Autodesk Inventor part; units mm, degrees
(part 2 of 2)
  spline S152 degree 2 poles (85.5825, 374.6714) (85.5825, 373.4202) (84.1936, 371.3057) (81.7162, 370.2172) (79.8144, 370.2172) knots 0 0 0 1 2 3 3 3 projected
  spline S153 degree 2 poles (79.8144, 370.2172) (76.4987, 370.2172) (73.9338, 372.7696) (73.7711, 374.7465) knots 0 0 0 1 2 2 2 projected
  line L321 (73.7711, 374.7465) -> (77.5998, 374.9842) projected
  spline S154 degree 2 poles (65.5507, 383.6676) (68.7913, 383.6676) (72.3072, 380.1767) (72.3072, 377.0362) knots 0 0 0 1 2 2 2 projected
  spline S155 degree 2 poles (72.3072, 377.0362) (72.3072, 374.759) (70.7682, 371.8437) (67.8654, 370.2172) (65.7008, 370.2172) knots 0 0 0 1 2 3 3 3 projected
  spline S156 degree 2 poles (65.7008, 370.2172) (63.5112, 370.2172) (60.621, 371.6185) (58.8317, 374.6589) (58.8317, 376.9361) knots 0 0 0 1 2 3 3 3 projected
  spline S157 degree 2 poles (58.8317, 376.9361) (58.8317, 380.1142) (62.3852, 383.6676) (65.5507, 383.6676) knots 0 0 0 1 2 2 2 projected
  line L322 (35.6094, 377.8495) -> (41.8154, 377.8495) projected
  line L323 (41.8154, 377.8495) -> (41.8154, 372.3192) projected
  spline S158 degree 2 poles (41.8154, 372.3192) (40.0262, 371.093) (37.286, 370.2172) (35.4092, 370.2172) knots 0 0 0 1 2 2 2 projected
  spline S159 degree 2 poles (35.4092, 370.2172) (33.0945, 370.2172) (30.1667, 371.7937) (28.5651, 374.9217) (28.5651, 376.9486) knots 0 0 0 1 2 3 3 3 projected
  spline S160 degree 2 poles (28.5651, 376.9486) (28.5651, 379.0757) (30.3168, 382.2162) (32.0185, 383.042) knots 0 0 0 1 2 2 2 projected
  spline S161 degree 2 poles (32.0185, 383.042) (33.3447, 383.6676) (35.5719, 383.6676) knots 0 0 0 1 1 1 projected
  spline S162 degree 2 poles (35.5719, 383.6676) (37.7365, 383.6676) (39.876, 382.8918) (41.2899, 381.2403) (41.6402, 379.9891) knots 0 0 0 1 2 3 3 3 projected
  line L324 (41.6402, 379.9891) -> (37.7615, 379.2884) projected
  spline S163 degree 2 poles (37.7615, 379.2884) (37.5238, 380.0266) (36.3726, 380.8148) (35.4843, 380.8148) knots 0 0 0 1 2 2 2 projected
  spline S164 degree 2 poles (35.4843, 380.8148) (34.1705, 380.8148) (32.594, 378.9756) (32.594, 376.9862) knots 0 0 0 1 2 2 2 projected
  spline S165 degree 2 poles (32.594, 376.9862) (32.594, 374.8841) (34.183, 373.0699) (35.6094, 373.0699) knots 0 0 0 1 2 2 2 projected
  spline S166 degree 2 poles (35.6094, 373.0699) (36.2851, 373.0699) (37.5112, 373.4578) (38.2995, 373.9332) knots 0 0 0 1 2 2 2 projected
  line L325 (38.2995, 373.9332) -> (38.2995, 375.1469) projected
  line L326 (38.2995, 375.1469) -> (35.6094, 375.1469) projected
  line L327 (35.6094, 375.1469) -> (35.6094, 377.8495) projected
  line L328 (8.9212, 383.4424) -> (15.6152, 383.4424) projected
  spline S167 degree 2 poles (15.6152, 383.4424) (17.467, 383.4424) (19.4439, 382.8043) (20.645, 381.0776) (20.645, 379.8389) knots 0 0 0 1 2 3 3 3 projected
  spline S168 degree 2 poles (20.645, 379.8389) (20.645, 378.7504) (19.7191, 377.1864) (18.9184, 376.6984) knots 0 0 0 1 2 2 2 projected
  spline S169 degree 2 poles (18.9184, 376.6984) (18.4054, 376.3856) (17.5045, 376.1854) knots 0 0 0 1 1 1 projected
  spline S170 degree 2 poles (17.5045, 376.1854) (18.2177, 375.9477) (18.5555, 375.7099) knots 0 0 0 1 1 1 projected
  spline S171 degree 2 poles (18.5555, 375.7099) (18.7682, 375.5473) (19.6065, 374.4963) (19.7567, 374.2085) knots 0 0 0 1 2 2 2 projected
  line L329 (19.7567, 374.2085) -> (21.696, 370.4424) projected
  line L330 (21.696, 370.4424) -> (17.1542, 370.4424) projected
  line L331 (17.1542, 370.4424) -> (15.0146, 374.4212) projected
  spline S172 degree 2 poles (15.0146, 374.4212) (14.6142, 375.1844) (14.3014, 375.4222) knots 0 0 0 1 1 1 projected
  spline S173 degree 2 poles (14.3014, 375.4222) (13.8635, 375.7225) (13.313, 375.7225) knots 0 0 0 1 1 1 projected
  line L332 (13.313, 375.7225) -> (12.9626, 375.7225) projected
  line L333 (12.9626, 375.7225) -> (12.9626, 370.4424) projected
  line L334 (12.9626, 370.4424) -> (8.9212, 370.4424) projected
  line L335 (8.9212, 370.4424) -> (8.9212, 383.4424) projected
  line L336 (-1.8516, 372.5944) -> (-2.4897, 370.4424) projected
  line L337 (-2.4897, 370.4424) -> (-6.5937, 370.4424) projected
  line L338 (-6.5937, 370.4424) -> (-1.7015, 383.4424) projected
  line L339 (-1.7015, 383.4424) -> (2.6903, 383.4424) projected
  line L340 (2.6903, 383.4424) -> (7.5699, 370.4424) projected
  line L341 (7.5699, 370.4424) -> (3.3659, 370.4424) projected
  line L342 (3.3659, 370.4424) -> (2.7153, 372.5944) projected
  line L343 (2.7153, 372.5944) -> (-1.8516, 372.5944) projected
  spline S174 degree 2 poles (-25.0114, 383.4424) (-23.1346, 383.4424) (-21.1201, 381.5781) (-21.1201, 380.2018) knots 0 0 0 1 2 2 2 projected
  spline S175 degree 2 poles (-21.1201, 380.2018) (-21.1201, 379.0507) (-21.8333, 378.2249) knots 0 0 0 1 1 1 projected
  spline S176 degree 2 poles (-21.8333, 378.2249) (-22.3213, 377.6743) (-23.2472, 377.349) knots 0 0 0 1 1 1 projected
  spline S177 degree 2 poles (-23.2472, 377.349) (-21.8458, 377.0112) (-20.5196, 375.3721) (-20.5196, 374.1334) knots 0 0 0 1 2 2 2 projected
  spline S178 degree 2 poles (-20.5196, 374.1334) (-20.5196, 373.1325) (-21.458, 371.5184) (-22.2712, 371.043) knots 0 0 0 1 2 2 2 projected
  spline S179 degree 2 poles (-22.2712, 371.043) (-22.7842, 370.7552) (-23.7977, 370.6175) knots 0 0 0 1 1 1 projected
  spline S180 degree 2 poles (-23.7977, 370.6175) (-25.1615, 370.4424) (-25.5994, 370.4424) knots 0 0 0 1 1 1 projected
  line L344 (-25.5994, 370.4424) -> (-32.5311, 370.4424) projected
  line L345 (-32.5311, 370.4424) -> (-32.5311, 383.4424) projected
  line L346 (-32.5311, 383.4424) -> (-25.0114, 383.4424) projected
  line L347 (-65.0999, 383.4424) -> (-60.1952, 376.248) projected
  line L348 (-60.1952, 376.248) -> (-60.1952, 383.4424) projected
  line L349 (-60.1952, 383.4424) -> (-56.4041, 383.4424) projected
  line L350 (-56.4041, 383.4424) -> (-56.4041, 370.4424) projected
  line L351 (-56.4041, 370.4424) -> (-60.1952, 370.4424) projected
  line L352 (-60.1952, 370.4424) -> (-65.0749, 377.5993) projected
  line L353 (-65.0749, 377.5993) -> (-65.0749, 370.4424) projected
  line L354 (-65.0749, 370.4424) -> (-68.8535, 370.4424) projected
  line L355 (-68.8535, 370.4424) -> (-68.8535, 383.4424) projected
  line L356 (-68.8535, 383.4424) -> (-65.0999, 383.4424) projected
  line L357 (-86.9334, 383.4424) -> (-84.3184, 379.0632) projected
  line L358 (-84.3184, 379.0632) -> (-81.6909, 383.4424) projected
  line L359 (-81.6909, 383.4424) -> (-77.2491, 383.4424) projected
  line L360 (-77.2491, 383.4424) -> (-82.304, 375.8851) projected
  line L361 (-82.304, 375.8851) -> (-82.304, 370.4424) projected
  line L362 (-82.304, 370.4424) -> (-86.3328, 370.4424) projected
  line L363 (-86.3328, 370.4424) -> (-86.3328, 375.8851) projected
  line L364 (-86.3328, 375.8851) -> (-91.4002, 383.4424) projected
  line L365 (-91.4002, 383.4424) -> (-86.9334, 383.4424) projected
  line L366 (-104.3877, 383.4424) -> (-104.3877, 380.6522) projected
  line L367 (-104.3877, 380.6522) -> (-110.2684, 380.6522) projected
  line L368 (-110.2684, 380.6522) -> (-110.2684, 378.3875) projected
  line L369 (-110.2684, 378.3875) -> (-105.251, 378.3875) projected
  line L370 (-105.251, 378.3875) -> (-105.251, 375.76) projected
  line L371 (-105.251, 375.76) -> (-110.2684, 375.76) projected
  line L372 (-110.2684, 375.76) -> (-110.2684, 370.4424) projected
  line L373 (-110.2684, 370.4424) -> (-114.3097, 370.4424) projected
  line L374 (-114.3097, 370.4424) -> (-114.3097, 383.4424) projected
  line L375 (-114.3097, 383.4424) -> (-104.3877, 383.4424) projected
  line L376 (-98.1942, 383.4424) -> (-98.1942, 373.6455) projected
  line L377 (-98.1942, 373.6455) -> (-91.9257, 373.6455) projected
  line L378 (-91.9257, 373.6455) -> (-91.9257, 370.4424) projected
  line L379 (-91.9257, 370.4424) -> (-102.2106, 370.4424) projected
  line L380 (-102.2106, 370.4424) -> (-102.2106, 383.4424) projected
  line L381 (-102.2106, 383.4424) -> (-98.1942, 383.4424) projected
  line L382 (-71.7563, 383.4424) -> (-71.7563, 370.4424) projected
  line L383 (-71.7563, 370.4424) -> (-75.7852, 370.4424) projected
  line L384 (-75.7852, 370.4424) -> (-75.7852, 383.4424) projected
  line L385 (-75.7852, 383.4424) -> (-71.7563, 383.4424) projected
  line L386 (-47.1827, 377.8495) -> (-40.9767, 377.8495) projected
  line L387 (-40.9767, 377.8495) -> (-40.9767, 372.3192) projected
  spline S181 degree 2 poles (-40.9767, 372.3192) (-42.7659, 371.093) (-45.5061, 370.2172) (-47.3829, 370.2172) knots 0 0 0 1 2 2 2 projected
  spline S182 degree 2 poles (-47.3829, 370.2172) (-49.6976, 370.2172) (-52.6254, 371.7937) (-54.227, 374.9217) (-54.227, 376.9486) knots 0 0 0 1 2 3 3 3 projected
  spline S183 degree 2 poles (-54.227, 376.9486) (-54.227, 379.0757) (-52.4753, 382.2162) (-50.7736, 383.042) knots 0 0 0 1 2 2 2 projected
  spline S184 degree 2 poles (-50.7736, 383.042) (-49.4474, 383.6676) (-47.2202, 383.6676) knots 0 0 0 1 1 1 projected
  spline S185 degree 2 poles (-47.2202, 383.6676) (-45.0557, 383.6676) (-42.9161, 382.8918) (-41.5022, 381.2403) (-41.1519, 379.9891) knots 0 0 0 1 2 3 3 3 projected
  line L388 (-41.1519, 379.9891) -> (-45.0306, 379.2884) projected
  spline S186 degree 2 poles (-45.0306, 379.2884) (-45.2684, 380.0266) (-46.4195, 380.8148) (-47.3078, 380.8148) knots 0 0 0 1 2 2 2 projected
  spline S187 degree 2 poles (-47.3078, 380.8148) (-48.6216, 380.8148) (-50.1981, 378.9756) (-50.1981, 376.9862) knots 0 0 0 1 2 2 2 projected
  spline S188 degree 2 poles (-50.1981, 376.9862) (-50.1981, 374.8841) (-48.6091, 373.0699) (-47.1827, 373.0699) knots 0 0 0 1 2 2 2 projected
  spline S189 degree 2 poles (-47.1827, 373.0699) (-46.507, 373.0699) (-45.2809, 373.4578) (-44.4926, 373.9332) knots 0 0 0 1 2 2 2 projected
  line L389 (-44.4926, 373.9332) -> (-44.4926, 375.1469) projected
  line L390 (-44.4926, 375.1469) -> (-47.1827, 375.1469) projected
  line L391 (-47.1827, 375.1469) -> (-47.1827, 377.8495) projected
  line L392 (-7.6447, 383.4424) -> (-7.6447, 380.6647) projected
  line L393 (-7.6447, 380.6647) -> (-14.3762, 380.6647) projected
  line L394 (-14.3762, 380.6647) -> (-14.3762, 378.6002) projected
  line L395 (-14.3762, 378.6002) -> (-8.1326, 378.6002) projected
  line L396 (-8.1326, 378.6002) -> (-8.1326, 375.9477) projected
  line L397 (-8.1326, 375.9477) -> (-14.3762, 375.9477) projected
  line L398 (-14.3762, 375.9477) -> (-14.3762, 373.3827) projected
  line L399 (-14.3762, 373.3827) -> (-7.4445, 373.3827) projected
  line L400 (-7.4445, 373.3827) -> (-7.4445, 370.4424) projected
  line L401 (-7.4445, 370.4424) -> (-18.405, 370.4424) projected
  line L402 (-18.405, 370.4424) -> (-18.405, 383.4424) projected
  line L403 (-18.405, 383.4424) -> (-7.6447, 383.4424) projected
  line L404 (48.234, 383.4424) -> (48.234, 378.888) projected
  line L405 (48.234, 378.888) -> (52.6258, 378.888) projected
  line L406 (52.6258, 378.888) -> (52.6258, 383.4424) projected
  line L407 (52.6258, 383.4424) -> (56.6672, 383.4424) projected
  line L408 (56.6672, 383.4424) -> (56.6672, 370.4424) projected
  line L409 (56.6672, 370.4424) -> (52.6258, 370.4424) projected
  line L410 (52.6258, 370.4424) -> (52.6258, 375.6974) projected
  line L411 (52.6258, 375.6974) -> (48.234, 375.6974) projected
  line L412 (48.234, 375.6974) -> (48.234, 370.4424) projected
  line L413 (48.234, 370.4424) -> (44.2177, 370.4424) projected
  line L414 (44.2177, 370.4424) -> (44.2177, 383.4424) projected
  line L415 (44.2177, 383.4424) -> (48.234, 383.4424) projected
  line L416 (98.9078, 383.4424) -> (98.9078, 380.2268) projected
  line L417 (98.9078, 380.2268) -> (94.8038, 380.2268) projected
  line L418 (94.8038, 380.2268) -> (94.8038, 370.4424) projected
  line L419 (94.8038, 370.4424) -> (90.7875, 370.4424) projected
  line L420 (90.7875, 370.4424) -> (90.7875, 380.2268) projected
  line L421 (90.7875, 380.2268) -> (86.6835, 380.2268) projected
  line L422 (86.6835, 380.2268) -> (86.6835, 383.4424) projected
  line L423 (86.6835, 383.4424) -> (98.9078, 383.4424) projected
  line L424 (-157.35, 534) -> (-154.35, 534)
  line L425 (-1.5, 534) -> (1.5, 534)
  line L426 (154.35, 534) -> (157.35, 534)
  line L427 (-155.85, 534) -> (-155.85, 541) construction
  line L428 (-155.85, 541) -> (155.85, 541) construction
  circle A126 centre (-155.85, 541) radius 1.55
  line L429 (0, 534) -> (0, 541) construction
  line L430 (155.85, 534) -> (155.85, 541) construction
  circle A127 centre (0, 541) radius 1.55
  circle A128 centre (155.85, 541) radius 1.55
  line L431 (-116.7, 538) -> (-116.8, 538)
  line L432 (-116.8, 538) -> (-116.8, 534)
  line L433 (-116.8, 534) -> (-116.7, 534)
  line L434 (-116.7, 534) -> (-116.7, 538)
  line L435 (-39.3, 538) -> (-39.2, 538)
  line L436 (-39.2, 538) -> (-39.2, 534)
  line L437 (-39.2, 534) -> (-39.3, 534)
  line L438 (-39.3, 534) -> (-39.3, 538)
  line L439 (39.3, 538) -> (39.2, 538)
  line L440 (39.2, 538) -> (39.2, 534)
  line L441 (39.2, 534) -> (39.3, 534)
  line L442 (39.3, 534) -> (39.3, 538)
  line L443 (116.7, 538) -> (116.8, 538)
  line L444 (116.8, 538) -> (116.8, 534)
  line L445 (116.8, 534) -> (116.7, 534)
  line L446 (116.7, 534) -> (116.7, 538)
  point P0 (0, 0)
  dimension "d7" = 4
  dimension "d8" = 5
  dimension "d9" = 1.05
  dimension "d10" = 8.5
  dimension "d11" = 5
  dimension "d12" = 2.45
  dimension "d13" = 1.05
  dimension "d14" = 250
  dimension "d15" = 7
  dimension "d16" = 3.1
  dimension "d17" = 3.1
  dimension "d18" = 3.1
  dimension "d21" = 0.1
  dimension "d22" = 0.1
  dimension "d23" = 0.1
  dimension "d24" = 0.1
  constraints: 136 end point, 19 collinear, 10 parallel, 5 horizontal, 4 midpoint, 4 perpendicular, 3 centre point, 3 coincident, 2 point on line, 1 vertical
  measures "d7" distance between parallel lines of L49 L51
  measures "d8" distance between parallel lines of L53 L1
  measures "d9" distance between parallel lines of L5 L3
  measures "d10" distance between parallel lines of L11 L5
  measures "d11" distance between parallel lines of L39 L37
  measures "d12" distance between parallel lines of L39 L41
  measures "d13" distance between parallel lines of L41 L43
  measures "d14" distance between parallel lines of L263 L51
  measures "d15" distance between parallel lines of L227 L428
  measures "d16" diameter of A126
  measures "d17" diameter of A127
  measures "d18" diameter of A128
  measures "d21" distance between parallel lines of L434 L432
  measures "d22" distance between parallel lines of L224 L436
  measures "d23" distance between parallel lines of L442 L440
  measures "d24" distance between parallel lines of L262 L444
extrude "Выдавливание1" add sketch "Эскиз1" against normal blind 4 contours L53 L52 L51 L50 L49 L48 L47 L46 L45 L44 L43 L42 L41 L40 L39 L38 L37 L36 L249 L426 L261 L444 L443 L263 L439 L440 L265 L425 L223 L436 L435 L225 L431 L432 L227 L424 L239 L28 L27 L26 L25 L24 L23 L22 L21 L20 L19 L18 L17 L16 L15 L14 L13 L12 L11 L10 L9 L8 L7 L6 L5 L4 L3 L2 L1 L0 | L261 L262 L443 L444 | L264 L265 L440 L439 | L223 L224 L435 L436 | L432 L431 L226 L227
extrude "Выдавливание2" cut sketch "Эскиз1" against normal blind 4 contours L261 L262 L443 L444 | L264 L265 L440 L439 | L223 L224 L435 L436 | L432 L431 L226 L227
sketch "Эскиз2" plane through (0, 0, 0) normal (0, 0, 1) x (1, 0, 0)
  line L0 (195, 714) -> (195, 604) projected
  line L1 (195, 714) -> (191, 714) projected
  line L2 (191, 604) -> (191, 714) projected
  line L3 (195, 604) -> (191, 604) projected
  line L4 (-191, 714) -> (-191, 604) projected
  line L5 (-191, 714) -> (-195, 714) projected
  line L6 (-195, 604) -> (-195, 714) projected
  line L7 (-191, 604) -> (-195, 604) projected
  line L8 (-195, 784) -> (-195, 534) projected
  line L9 (-191, 714) -> (-195, 714)
  line L10 (-195, 714) -> (-195, 714.1)
  line L11 (-195, 714.1) -> (-191, 714.1)
  line L12 (-191, 714.1) -> (-191, 714)
  line L13 (-191, 604) -> (-195, 604)
  line L14 (-195, 604) -> (-195, 603.9)
  line L15 (-195, 603.9) -> (-191, 603.9)
  line L16 (-191, 603.9) -> (-191, 604)
  line L17 (191, 604) -> (195, 604)
  line L18 (195, 604) -> (195, 603.9)
  line L19 (195, 603.9) -> (191, 603.9)
  line L20 (191, 603.9) -> (191, 604)
  line L21 (195, 784) -> (195, 534) projected
  line L22 (191, 714) -> (195, 714)
  line L23 (195, 714) -> (195, 714.1)
  line L24 (195, 714.1) -> (191, 714.1)
  line L25 (191, 714.1) -> (191, 714)
  point P0 (0, 0)
  dimension "d27" = 0.1
  dimension "d28" = 0.1
  dimension "d29" = 0.1
  dimension "d30" = 0.1
  constraints: 32 end point, 8 parallel, 4 horizontal, 4 perpendicular, 3 point on line
  measures "d27" distance between parallel lines of L5 L11
  measures "d28" distance between parallel lines of L15 L13
  measures "d29" distance between parallel lines of L19 L17
  measures "d30" distance between parallel lines of L1 L24
extrude "Выдавливание3" cut sketch "Эскиз2" against normal blind 4
sketch "Эскиз3" plane through (0, 0, 0) normal (0, 0, 1) x (1, 0, 0)
  line L0 (191, 714.1) -> (195, 714.1)
  line L1 (195, 714.1) -> (195, 784)
  line L2 (195, 784) -> (157.35, 784)
  line L3 (157.35, 784) -> (157.35, 779)
  line L4 (157.35, 779) -> (158.65, 779)
  line L5 (158.65, 779) -> (158.65, 776.55)
  line L6 (158.65, 776.55) -> (157.35, 776.55)
  line L7 (157.35, 776.55) -> (157.35, 775.5)
  line L8 (157.35, 775.5) -> (154.35, 775.5)
  line L9 (154.35, 775.5) -> (154.35, 776.55)
  line L10 (154.35, 776.55) -> (153.05, 776.55)
  line L11 (153.05, 776.55) -> (153.05, 779)
  line L12 (153.05, 779) -> (154.35, 779)
  line L13 (154.35, 779) -> (154.35, 784)
  line L14 (154.35, 784) -> (116.7, 784)
  line L15 (116.7, 784) -> (116.7, 788)
  line L16 (116.7, 788) -> (39.3, 788)
  line L17 (39.3, 788) -> (39.3, 784)
  line L18 (39.3, 784) -> (1.5, 784)
  line L19 (1.5, 784) -> (1.5, 779)
  line L20 (1.5, 779) -> (2.8, 779)
  line L21 (2.8, 779) -> (2.8, 776.55)
  line L22 (2.8, 776.55) -> (1.5, 776.55)
  line L23 (1.5, 776.55) -> (1.5, 775.5)
  line L24 (1.5, 775.5) -> (-1.5, 775.5)
  line L25 (-1.5, 775.5) -> (-1.5, 776.55)
  line L26 (-1.5, 776.55) -> (-2.8, 776.55)
  line L27 (-2.8, 776.55) -> (-2.8, 779)
  line L28 (-2.8, 779) -> (-1.5, 779)
  line L29 (-1.5, 779) -> (-1.5, 784)
  line L30 (-1.5, 784) -> (-39.3, 784)
  line L31 (-39.3, 784) -> (-39.3, 788)
  line L32 (-39.3, 788) -> (-116.7, 788)
  line L33 (-116.7, 788) -> (-116.7, 784)
  line L34 (-116.7, 784) -> (-154.35, 784)
  line L35 (-154.35, 784) -> (-154.35, 779)
  line L36 (-154.35, 779) -> (-153.05, 779)
  line L37 (-153.05, 779) -> (-153.05, 776.55)
  line L38 (-153.05, 776.55) -> (-154.35, 776.55)
  line L39 (-154.35, 776.55) -> (-154.35, 775.5)
  line L40 (-154.35, 775.5) -> (-157.35, 775.5)
  line L41 (-157.35, 775.5) -> (-157.35, 776.55)
  line L42 (-157.35, 776.55) -> (-158.65, 776.55)
  line L43 (-158.65, 776.55) -> (-158.65, 779)
  line L44 (-158.65, 779) -> (-157.35, 779)
  line L45 (-157.35, 779) -> (-157.35, 784)
  line L46 (-157.35, 784) -> (-195, 784)
  line L47 (-195, 784) -> (-195, 714.1)
  line L48 (-195, 714.1) -> (-191, 714.1)
  line L49 (-191, 714.1) -> (-191, 603.9)
  line L50 (-191, 603.9) -> (-195, 603.9)
  line L51 (-195, 603.9) -> (-195, 534)
  line L52 (-195, 534) -> (-116.8, 534)
  line L53 (-116.8, 534) -> (-116.8, 538)
  line L54 (-116.8, 538) -> (-39.2, 538)
  line L55 (-39.2, 538) -> (-39.2, 534)
  line L56 (-39.2, 534) -> (39.2, 534)
  line L57 (39.2, 534) -> (39.2, 538)
  line L58 (39.2, 538) -> (116.8, 538)
  line L59 (116.8, 538) -> (116.8, 534)
  line L60 (116.8, 534) -> (195, 534)
  line L61 (195, 534) -> (195, 603.9)
  line L62 (195, 603.9) -> (191, 603.9)
  line L63 (191, 603.9) -> (191, 714.1)
  circle A0 centre (155.85, 541) radius 1.55
  circle A1 centre (0, 541) radius 1.55
  circle A2 centre (-155.85, 541) radius 1.55
  line L64 (195, 567.5) -> (192.5, 567.5)
  line L65 (192.5, 570.5) -> (195, 570.5)
  line L66 (192.5, 750.5) -> (195, 750.5)
  line L67 (195, 747.5) -> (192.5, 747.5)
  line L68 (-195, 750.5) -> (-192.5, 750.5)
  line L69 (-192.5, 747.5) -> (-195, 747.5)
  line L70 (-195, 570.5) -> (-192.5, 570.5)
  line L71 (-192.5, 567.5) -> (-195, 567.5)
  line L72 (-191, 749) -> (-191, 749)
  line L73 (-191, 569) -> (-191, 569)
  line L74 (191, 569) -> (191, 569)
  line L75 (191, 749) -> (191, 749)
  arc A3 (192.5, 750.5) -> (191, 749) centre (192.5, 749) ccw
  arc A4 (191, 749) -> (192.5, 747.5) centre (192.5, 749) ccw
  arc A5 (192.5, 570.5) -> (191, 569) centre (192.5, 569) ccw
  arc A6 (191, 569) -> (192.5, 567.5) centre (192.5, 569) ccw
  arc A7 (-191, 569) -> (-192.5, 570.5) centre (-192.5, 569) ccw
  arc A8 (-192.5, 567.5) -> (-191, 569) centre (-192.5, 569) ccw
  arc A9 (-191, 749) -> (-192.5, 750.5) centre (-192.5, 749) ccw
  arc A10 (-192.5, 747.5) -> (-191, 749) centre (-192.5, 749) ccw
  point P0 (0, 0)
  dimension "d33" = 1.5
  constraints: 152 end point, 16 point on circle, 16 tangent, 14 centre point, 7 equal radius
  measures "d33" radius of A3
extrude "Выдавливание4" cut sketch "Эскиз3" against normal blind 4 contours L67 A4 A3 L66 L1 | L61 L64 A6 A5 L65 | L51 L70 A7 A8 L71 | L47 L68 A9 A10 L69
sketch "Эскиз4" plane through (0, 0, 0) normal (0, 0, 1) x (1, 0, 0)
  line L0 (-192.5, 747.5) -> (-195, 747.5) projected
  line L1 (-195, 747.5) -> (-195, 714.1) projected
  line L2 (-195, 714.1) -> (-191, 714.1) projected
  line L3 (-191, 714.1) -> (-191, 603.9) projected
  line L4 (-191, 603.9) -> (-195, 603.9) projected
  line L5 (-195, 603.9) -> (-195, 570.5) projected
  line L6 (-195, 570.5) -> (-192.5, 570.5) projected
  arc A0 (-192.5, 567.5) -> (-192.5, 570.5) centre (-192.5, 569) ccw projected
  line L7 (-192.5, 567.5) -> (-195, 567.5) projected
  line L8 (-195, 567.5) -> (-195, 534) projected
  line L9 (-195, 534) -> (-116.8, 534) projected
  line L10 (-116.8, 534) -> (-116.8, 538) projected
  line L11 (-116.8, 538) -> (-39.2, 538) projected
  line L12 (-39.2, 538) -> (-39.2, 534) projected
  line L13 (-39.2, 534) -> (39.2, 534) projected
  line L14 (39.2, 534) -> (39.2, 538) projected
  line L15 (39.2, 538) -> (116.8, 538) projected
  line L16 (116.8, 538) -> (116.8, 534) projected
  line L17 (116.8, 534) -> (195, 534) projected
  line L18 (195, 534) -> (195, 567.5) projected
  line L19 (195, 567.5) -> (192.5, 567.5) projected
  arc A1 (192.5, 570.5) -> (192.5, 567.5) centre (192.5, 569) ccw projected
  line L20 (192.5, 570.5) -> (195, 570.5) projected
  line L21 (195, 570.5) -> (195, 603.9) projected
  line L22 (195, 603.9) -> (191, 603.9) projected
  line L23 (191, 603.9) -> (191, 714.1) projected
  line L24 (191, 714.1) -> (195, 714.1) projected
  line L25 (195, 714.1) -> (195, 747.5) projected
  line L26 (195, 747.5) -> (192.5, 747.5) projected
  arc A2 (192.5, 750.5) -> (192.5, 747.5) centre (192.5, 749) ccw projected
  line L27 (192.5, 750.5) -> (195, 750.5) projected
  line L28 (195, 750.5) -> (195, 784) projected
  line L29 (195, 784) -> (157.35, 784) projected
  line L30 (157.35, 784) -> (157.35, 779) projected
  line L31 (157.35, 779) -> (158.65, 779) projected
  line L32 (158.65, 779) -> (158.65, 776.55) projected
  line L33 (158.65, 776.55) -> (157.35, 776.55) projected
  line L34 (157.35, 776.55) -> (157.35, 775.5) projected
  line L35 (157.35, 775.5) -> (154.35, 775.5) projected
  line L36 (154.35, 775.5) -> (154.35, 776.55) projected
  line L37 (154.35, 776.55) -> (153.05, 776.55) projected
  line L38 (153.05, 776.55) -> (153.05, 779) projected
  line L39 (153.05, 779) -> (154.35, 779) projected
  line L40 (154.35, 779) -> (154.35, 784) projected
  line L41 (154.35, 784) -> (116.7, 784) projected
  line L42 (116.7, 784) -> (116.7, 788) projected
  line L43 (116.7, 788) -> (39.3, 788) projected
  line L44 (39.3, 788) -> (39.3, 784) projected
  line L45 (39.3, 784) -> (1.5, 784) projected
  line L46 (1.5, 784) -> (1.5, 779) projected
  line L47 (1.5, 779) -> (2.8, 779) projected
  line L48 (2.8, 779) -> (2.8, 776.55) projected
  line L49 (2.8, 776.55) -> (1.5, 776.55) projected
  line L50 (1.5, 776.55) -> (1.5, 775.5) projected
  line L51 (1.5, 775.5) -> (-1.5, 775.5) projected
  line L52 (-1.5, 775.5) -> (-1.5, 776.55) projected
  line L53 (-1.5, 776.55) -> (-2.8, 776.55) projected
  line L54 (-2.8, 776.55) -> (-2.8, 779) projected
  line L55 (-2.8, 779) -> (-1.5, 779) projected
  line L56 (-1.5, 779) -> (-1.5, 784) projected
  line L57 (-1.5, 784) -> (-39.3, 784) projected
  line L58 (-39.3, 784) -> (-39.3, 788) projected
  line L59 (-39.3, 788) -> (-116.7, 788) projected
  line L60 (-116.7, 788) -> (-116.7, 784) projected
  line L61 (-116.7, 784) -> (-154.35, 784) projected
  line L62 (-154.35, 784) -> (-154.35, 779) projected
  line L63 (-154.35, 779) -> (-153.05, 779) projected
  line L64 (-153.05, 779) -> (-153.05, 776.55) projected
  line L65 (-153.05, 776.55) -> (-154.35, 776.55) projected
  line L66 (-154.35, 776.55) -> (-154.35, 775.5) projected
  line L67 (-154.35, 775.5) -> (-157.35, 775.5) projected
  line L68 (-157.35, 775.5) -> (-157.35, 776.55) projected
  line L69 (-157.35, 776.55) -> (-158.65, 776.55) projected
  line L70 (-158.65, 776.55) -> (-158.65, 779) projected
  line L71 (-158.65, 779) -> (-157.35, 779) projected
  line L72 (-157.35, 779) -> (-157.35, 784) projected
  line L73 (-157.35, 784) -> (-195, 784) projected
  line L74 (-195, 784) -> (-195, 750.5) projected
  line L75 (-195, 750.5) -> (-192.5, 750.5) projected
  arc A3 (-192.5, 747.5) -> (-192.5, 750.5) centre (-192.5, 749) ccw projected
  circle A4 centre (155.85, 541) radius 1.55 projected
  circle A5 centre (0, 541) radius 1.55 projected
  circle A6 centre (-155.85, 541) radius 1.55 projected
  line L76 (191, 603.9) -> (191, 714.1) projected
  line L77 (191, 659) -> (182, 659) construction
  line L78 (-191, 603.9) -> (-191, 714.1) projected
  line L79 (-191, 659) -> (-173, 659) construction
  line L80 (-191, 660.5) -> (-186, 660.5)
  line L81 (-186, 660.5) -> (-186, 657.5)
  line L82 (-186, 657.5) -> (-191, 657.5)
  line L83 (-191, 657.5) -> (-191, 660.5)
  line L84 (-186, 661.8) -> (-183.55, 661.8)
  line L85 (-183.55, 661.8) -> (-183.55, 656.2)
  line L86 (-183.55, 656.2) -> (-186, 656.2)
  line L87 (-186, 656.2) -> (-186, 661.8)
  line L88 (-183.55, 660.5) -> (-182.5, 660.5)
  line L89 (-182.5, 660.5) -> (-182.5, 657.5)
  line L90 (-182.5, 657.5) -> (-183.55, 657.5)
  line L91 (-183.55, 657.5) -> (-183.55, 660.5)
  line L92 (191, 660.5) -> (183.55, 660.5)
  line L93 (183.55, 660.5) -> (183.55, 657.5)
  line L94 (183.55, 657.5) -> (191, 657.5)
  line L95 (191, 657.5) -> (191, 660.5)
  line L96 (183.55, 661.8) -> (186, 661.8)
  line L97 (186, 661.8) -> (186, 656.2)
  line L98 (186, 656.2) -> (183.55, 656.2)
  line L99 (183.55, 656.2) -> (183.55, 661.8)
  line L100 (186, 660.5) -> (182.5, 660.5)
  line L101 (182.5, 660.5) -> (182.5, 657.5)
  line L102 (182.5, 657.5) -> (186, 657.5)
  line L103 (186, 657.5) -> (186, 660.5)
  point P0 (0, 0)
  dimension "d36" = 2.45
  dimension "d37" = 8.5
  dimension "d38" = 3
  dimension "d39" = 5.6
  dimension "d40" = 3
  dimension "d41" = 3
  dimension "d42" = 5.6
  dimension "d43" = 2.45
  dimension "d44" = 7.45
  dimension "d45" = 7.45
  dimension "d46" = 8.5
  dimension "d47" = 7.45
  dimension "d48" = 8.5
  dimension "d50" = 2.45
  constraints: 52 end point, 13 point on line, 12 parallel, 8 horizontal, 6 perpendicular, 2 midpoint, 3 other
  measures "d36" distance between parallel lines of L31 L33
  measures "d37" distance between parallel lines of L29 L35
  measures "d38" distance between parallel lines of L36 L34
  measures "d39" distance between parallel lines of L32 L38
  measures "d40" distance between parallel lines of L102 L100
  measures "d41" distance between parallel lines of L82 L80
  measures "d42" distance between parallel lines of L98 L96
  measures "d43" distance of L84.start L84.end
  measures "d44" distance between parallel lines of L41 L37
  measures "d45" distance between parallel lines of L3 L85
  measures "d46" distance between parallel lines of L3 L89
  measures "d47" distance between parallel lines of L23 L93
  measures "d48" distance between parallel lines of L23 L101
  measures "d50" distance between parallel lines of L97 L99
extrude "Выдавливание5" cut sketch "Эскиз4" against normal blind 4 contours L80 L81 L82 L3 | L87 L84 L85 L86 L81 | L88 L89 L90 L85 | L94 L97 L92 L23 | L97 L98 L99 L94 | L94 L93 L92 L97 | L92 L99 L96 L97 | L102 L101 L100 L93
